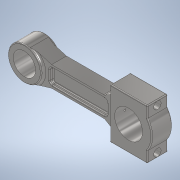
# Autodesk Inventor part: Шатун
Saved by Autodesk Inventor 2021 (Build 250183000, 183)
## iProperties
Created: 2020-11-29
Part Number: Шатун
Material: Сталь, углеродистая
Document SubType Name: Modeling
Designer: Тимоха
Mass: 29778 g
Surface Area: 3493.97 cm^2
Volume: 3793.38 cm^3
Density: 7.85 g/cm^3
Appearance: С умеренной полировкой
Author: Тимоха
Autodesk Inventor part; units mm, degrees
ref_plane "YZ Plane" through (0, 0, 0) normal (1, 0, 0) x (0, 1, 0)
ref_plane "XZ Plane" through (0, 0, 0) normal (0, 1, 0) x (-1, 0, 0)
ref_plane "XY Plane" through (0, 0, 0) normal (0, 0, 1) x (1, 0, 0)
sketch "Эскиз1" plane through (0, 0, 0) normal (0, 0, 1) x (1, 0, 0)
  circle A0 centre (0, 0) radius 60
  line L0 (0, 0) -> (560, 0)
  circle A1 centre (560, 0) radius 75
  circle A2 centre (0, 0) radius 90
  line L1 (560, 0) -> (560, 105)
  line L2 (560, 0) -> (560, -105)
  line L3 (560, 105) -> (460, 105)
  line L4 (560, 105) -> (660, 105)
  line L5 (560, -105) -> (460, -105)
  line L6 (560, -105) -> (660, -105)
  line L7 (560, 0) -> (660, 0)
  line L8 (660, 135) -> (660, -135)
  line L9 (460, 135) -> (460, -135)
  line L10 (460, 135) -> (660, 135)
  line L11 (460, -135) -> (660, -135)
  line L12 (660, 105) -> (660, 75)
  arc A3 (660, -75) -> (660, 75) centre (560, 0) ccw
  line L13 (71.239034, 55) -> (411.339746, 55)
  line L14 (71.239034, -55) -> (411.339746, -55)
  line L15 (460, 75) -> (450, 75)
  line L16 (450, 75) -> (418.839746, 57.009619)
  line L17 (460, -75) -> (450, -75)
  line L18 (450, -75) -> (418.839746, -57.009619)
  arc A4 (418.839746, -57.009619) -> (411.339746, -55) centre (411.339746, -70) ccw
  arc A5 (411.339746, 55) -> (418.839746, 57.009619) centre (411.339746, 70) ccw
  line L19 (25.607604, 86.280071) -> (131, 55)
  line L20 (25.607604, -86.280071) -> (131, -55)
  line L21 (131, 55) -> (131, 0)
  point P0 (460, 55)
  point P1 (460, -55)
  point P2 (415.358984, 55)
  point P3 (415.358984, -55)
  point P4 (460, -75)
  dimension "d0" = 120
  dimension "d1" = 560
  dimension "d2" = 150
  dimension "d3" = 180
  dimension "d4" = 105
  dimension "d5" = 105
  dimension "d6" = 100
  dimension "d7" = 100
  dimension "d11" = 100
  dimension "d12" = 270
  dimension "d13" = 30
  dimension "d14" = 55
  dimension "d15" = 110
  dimension "d17" = 30
  dimension "d18" = 10
  dimension "d19" = 15
  constraints: 44 end point, 12 point on line, 10 point on circle, 9 symmetric about line, 8 horizontal, 6 centre point, 5 tangent, 4 coincident, 3 vertical, 1 equal radius, 1 midpoint, 1 parallel, 1 perpendicular
  measures "d0" diameter of A0
  measures "d1" distance of L0.start L0.end
  measures "d2" diameter of A1
  measures "d3" diameter of A2
  measures "d4" distance of L1.start L1.end
  measures "d5" distance of L1.start L2.end
  measures "d6" distance of L1.end L3.end
  measures "d7" distance of L1.end L4.end
  measures "d11" distance of L7.end L1.start
  measures "d12" distance of L8.start L8.end
  measures "d13" distance of L12.end L4.end
  measures "d14" distance between parallel lines of L13 L0
  measures "d15" distance between parallel lines of L14 L13
  measures "d17" angle of L13 L16
  measures "d18" distance of L15.start L15.end
  measures "d19" radius of A4
extrude "Выдавливание1" add sketch "Эскиз1" along normal mid plane 110 contours A2 | L9 L3 L1 A1 L0 | L0 A1 L2 L5 L9 | L1 L4 L8 L7 A1 | A1 L7 L8 L6 L2 | L9 L10 L8 L4 L3 | L5 L6 L8 L11 L9 | L8 A3
extrude "Выдавливание2" add sketch "Эскиз1" along normal mid plane 80 contours A2 L13 L21 L0 | L0 L9 L17 L18 A4 L14 A2 | L21 L13 A5 L16 L15 L9 L0 | A2 L19 L13 | L14 L20 A2
sketch "Эскиз2" plane through (0, 0, -40) normal (0, 0, -1) x (-1, 0, 0)
  arc A0 (-418.839746, 57.009619) -> (-411.339746, 55) centre (-411.339746, 70) ccw
  line L0 (-418.839746, 57.009619) -> (-450, 75)
  line L1 (-450, 75) -> (-460, 75)
  line L2 (-460, -75) -> (-460, 75)
  line L3 (-460, -75) -> (-450, -75)
  line L4 (-450, -75) -> (-418.839746, -57.009619)
  arc A1 (-411.339746, -55) -> (-418.839746, -57.009619) centre (-411.339746, -70) ccw
  line L5 (-411.339746, -55) -> (-131, -55)
  line L6 (-131, -55) -> (-25.607604, -86.280071)
  arc A2 (-25.607604, 86.280071) -> (-25.607604, -86.280071) centre (0, 0) ccw
  line L7 (-25.607604, 86.280071) -> (-131, 55)
  line L8 (-131, 55) -> (-411.339746, 55)
  line L9 (-430, 0) -> (-430, 25)
  line L10 (-415, 40) -> (-135, 40)
  line L11 (-120, 25) -> (-120, 0)
  arc A3 (-415, 40) -> (-430, 25) centre (-415, 25) ccw
  arc A4 (-120, 25) -> (-135, 40) centre (-135, 25) ccw
  line L12 (0, 0) -> (-560, 0)
  line L13 (-430, 0) -> (-430, -25)
  line L14 (-415, -40) -> (-135, -40)
  line L15 (-120, -25) -> (-120, 0)
  arc A5 (-430, -25) -> (-415, -40) centre (-415, -25) ccw
  arc A6 (-135, -40) -> (-120, -25) centre (-135, -25) ccw
  point P0 (-430, 40)
  dimension "d24" = 40
  dimension "d25" = 15
  dimension "d40" = 430
  dimension "d44" = 310
  constraints: 12 end point, 8 point on circle, 6 symmetric about line, 4 centre point, 4 tangent, 2 perpendicular, 2 point on line, 1 equal radius, 1 vertical, 2 other
  measures "d24" distance of L9.start point (-430, 40)
  measures "d25" radius of A3
  measures "d40" distance from line of point (0, 0) L13
  measures "d44" distance between parallel lines of L11 L9
extrude "Выдавливание3" cut sketch "Эскиз2" against normal blind 20 contours L9 A3 L10 A4 L11 L12 | L12 L15 A6 L14 A5 L13
fillet "Сопряжение1" radius 5 8 edges at (124.3934, 35.6066, -20) (120, 0, -20) (124.3934, -35.6066, -20) (275, -40, -20) (425.6066, -35.6066, -20) (430, 0, -20) (425.6066, 35.6066, -20) (275, 40, -20)
mirror "Зеркальное отражение1" about plane through (0, 0, 0) normal (0, 0, 1) of "Выдавливание3", "Сопряжение1"
fillet "Сопряжение3" radius 5 16 edges at (124.3934, -35.6066, 40) (120, 0, 40) (124.3934, 35.6066, 40) (275, 40, 40) (425.6066, 35.6066, 40) (430, 0, 40) (425.6066, -35.6066, 40) (275, -40, 40) (124.3934, 35.6066, -40) (120, 0, -40) (124.3934, -35.6066, -40) (275, -40, -40) (425.6066, -35.6066, -40) (430, 0, -40) (425.6066, 35.6066, -40) (275, 40, -40)
sketch "Эскиз3" plane through (460, -135, 55) normal (-1, 0, 0) x (0, 0, 1)
  line L0 (-55, -54) -> (-55, 324) projected
  line L1 (-132, 135) -> (22, 135) projected
  line L2 (-55, 135) -> (-55, 25)
  line L3 (-55, 25) -> (-55, 245)
  circle A0 centre (-55, 25) radius 20
  circle A1 centre (-55, 245) radius 20
  dimension "d31" = 110
  dimension "d32" = 220
  dimension "d33" = 40
  dimension "d34" = 40
  constraints: 4 end point, 2 centre point, 2 coincident, 2 point on line
  measures "d31" distance of L2.start L2.end
  measures "d32" distance of L2.end L3.end
  measures "d33" diameter of A0
  measures "d34" diameter of A1
extrude "Выдавливание4" cut sketch "Эскиз3" against normal through all
fillet "Сопряжение4" radius 10 6 edges at (460, 0, 40) (460, 0, -40) (72.1273, 53.8299, 40) (72.1273, -53.8299, 40) (72.1273, -53.8299, -40) (72.1273, 53.8299, -40)
fillet "Сопряжение5" radius 5 18 edges at (685, 0, 55) (660, 105, 55) (560, 135, 55) (460, 0, 55) (560, -135, 55) (660, -105, 55) (685, 0, -55) (660, -105, -55) (560, -135, -55) (460, 0, -55) (560, 135, -55) (660, 105, -55) (660, -135, 0) (460, -135, 0) (660, 135, 0) (460, 135, 0) (-90, 0, 55) (-90, 0, -55)
sketch "Эскиз4" plane through (0, 0, 0) normal (1, 0, 0) x (0, 1, 0)
  circle A0 centre (0, 0) radius 5
  dimension "d41" = 10
  constraints: 1 centre point, 1 coincident
  measures "d41" diameter of A0
extrude "Выдавливание5" cut sketch "Эскиз4" along normal blind 520.25
